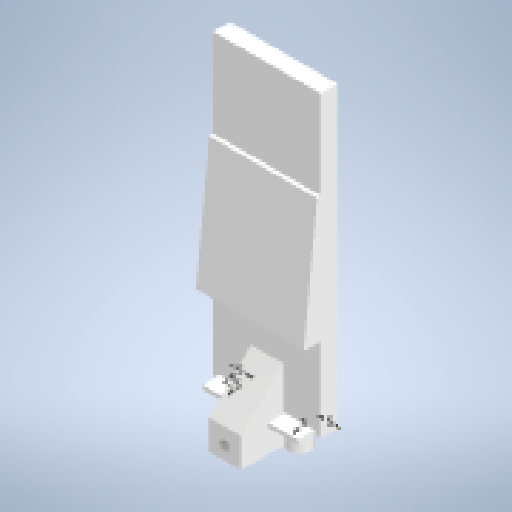
# Autodesk Inventor part: SchubstangeA
Saved by Autodesk Inventor 2025 (Build 290162010, 162A)
## iProperties
Created: 2024-11-26
Part Number: SchubstangeA
Material: PC/ABS-Kunststoff, 3DDruck, PLA
Document SubType Name: Modeling
Designer: Admin
Density: 1.1 g/cm^3
Appearance: Glatt - Weiß(2)
Author: Admin
Autodesk Inventor part; units mm, degrees
ref_plane "YZ Plane" through (0, 0, 0) normal (1, 0, 0) x (0, 1, 0)
ref_plane "XZ Plane" through (0, 0, 0) normal (0, 1, 0) x (-1, 0, 0)
ref_plane "XY Plane" through (0, 0, 0) normal (0, 0, 1) x (1, 0, 0)
sketch "Skizze1" plane through (0, 0, 0) normal (0, 1, 0) x (-1, 0, 0)
  line L0 (16.6592, -105.2226) -> (-8.9408, -105.2226)
  line L1 (-8.9408, -105.2226) -> (-8.9408, -28.2226)
  line L2 (16.6592, -28.2226) -> (16.6592, -105.2226)
  line L3 (3.8592, 157.3916) -> (3.8592, -262.6084)
  line L4 (16.6592, -28.2226) -> (-8.9408, -28.2226)
  line L5 (-8.9408, -105.2226) -> (0.0592, -105.2226)
  line L6 (0.0592, -105.2226) -> (0.0592, -99.2226)
  line L7 (0.0592, -99.2226) -> (-8.9408, -99.2226)
  line L8 (-8.9408, -99.2226) -> (-8.9408, -105.2226)
  line L9 (16.6592, -105.2226) -> (7.6592, -105.2226)
  line L10 (7.6592, -105.2226) -> (7.6592, -99.2226)
  line L11 (7.6592, -99.2226) -> (16.6592, -99.2226)
  line L12 (16.6592, -99.2226) -> (16.6592, -105.2226)
  point P0 (0, 0)
  point P1 (3.8592, -105.2226)
  point P2 (0.0592, -105.2226)
  point P3 (7.6592, -105.2226)
  dimension "d9" = 25.6
  dimension "d48" = 77
  dimension "d49" = 9
  dimension "d50" = 6
  dimension "d51" = 9
  dimension "d52" = 6
  constraints: 26 end point, 5 parallel, 3 horizontal, 3 perpendicular, 1 midpoint, 1 point on line, 1 vertical, 3 other
  measures "d9" distance of L0.start L0.end
  measures "d48" distance between parallel lines of L4 L0
  measures "d49" distance of L7.end L6.end
  measures "d50" distance of L6.end L5.end
  measures "d51" distance of L10.end L11.end
  measures "d52" distance of L9.end L10.end
extrude "Extrusion1" add sketch "Skizze1" along normal blind 4 contours L0 L3 L4 L2 L11 L10 | L0 L6 L7 L1 L4 L3
sketch "Skizze3" plane through (1.1408, 0, -99.2226) normal (0, 0, -1) x (-1, 0, 0)
  line L0 (-2.8, 4) -> (-2.8, 0)
  circle A0 centre (-2.8, 0) radius 2.5
  line L1 (12.8, 4) -> (12.8, 0)
  circle A1 centre (12.8, 0) radius 2.5
  line L2 (8.8, 4) -> (17.8, 4) projected
  line L3 (-7.8, 4) -> (1.2, 4) projected
  line L4 (-2.8, 0) -> (12.8, 0)
  dimension "d29" = 5
  dimension "d54" = 5
  dimension "d66" = 4
  dimension "d69" = 5
  dimension "d70" = 5
  constraints: 8 end point, 2 centre point, 2 point on line, 2 vertical, 1 horizontal
  measures "d29" diameter of A0
  measures "d54" diameter of A1
  measures "d66" distance from line of L1.end L2
  measures "d69" distance from line of L2.end L1
  measures "d70" distance from line of L3.start L0
extrude "Extrusion2" add sketch "Skizze3" along normal blind 4
sketch "Skizze4" plane through (0, 0, 0) normal (0, -1, 0) x (1, 0, 0)
  line L0 (8.9408, -28.2226) -> (8.9408, -99.2226) projected
  line L1 (-16.6592, -89.2226) -> (8.9408, -89.2226)
  line L2 (8.9408, -89.2226) -> (8.9408, -49.2226)
  line L3 (8.9408, -49.2226) -> (-16.6592, -49.2226)
  line L4 (-16.6592, -49.2226) -> (-16.6592, -89.2226)
  line L5 (-16.6592, -99.2226) -> (-16.6592, -28.2226) projected
  line L6 (-0.0592, -105.2226) -> (-7.6592, -105.2226) projected
  point P0 (0, 0)
  point P1 (8.9408, -89.2226)
  dimension "d34" = 40
  dimension "d57" = 16
  constraints: 8 end point, 2 parallel, 1 collinear, 1 horizontal, 1 perpendicular, 1 point on line
  measures "d34" distance of L2.end L1.end
  measures "d57" distance between parallel lines of L6 L1
extrude "Extrusion3" add sketch "Skizze4" along normal blind 5
chamfer "Fasen1" distance 40 distance2 4 1 edges at (-3.8592, -5, -49.2226) measured on face at (-3.8592, -5, -49.7226)
sketch "Skizze5" plane through (8.9408, 0, -89.2226) normal (0, 0, -1) x (-1, 0, 0)
  line L0 (0, 0) -> (25.6, 0) projected
  line L1 (0, 0) -> (0, -5) projected
  line L2 (25.6, -5) -> (0, -5) projected
  line L3 (25.6, 0) -> (25.6, -5) projected
  point P0 (8.9408, 0)
extrude "Extrusion4" cut sketch "Skizze5" against normal blind 10
sketch "Skizze6" plane through (0, 0, 0) normal (0, -1, 0) x (1, 0, 0)
  line L0 (-7.6592, -99.2226) -> (-16.6592, -99.2226) projected
  line L1 (-15.1592, -99.2226) -> (-8.1592, -99.2226)
  line L2 (-8.1592, -99.2226) -> (-8.1592, -98.2226)
  line L3 (-8.1592, -98.2226) -> (-15.1592, -98.2226)
  line L4 (-15.1592, -98.2226) -> (-15.1592, -99.2226)
  line L5 (8.9408, -99.2226) -> (-0.0592, -99.2226) projected
  line L6 (7.4408, -99.2226) -> (0.4408, -99.2226)
  line L7 (0.4408, -99.2226) -> (0.4408, -98.2226)
  line L8 (0.4408, -98.2226) -> (7.4408, -98.2226)
  line L9 (7.4408, -98.2226) -> (7.4408, -99.2226)
  line L10 (1.4408, -99.2226) -> (6.4408, -99.2226) projected
  line L11 (-14.1592, -99.2226) -> (-9.1592, -99.2226) projected
  point P0 (0, 0)
  point P1 (6.4408, -99.2226)
  point P2 (-9.1592, -99.2226)
  point P3 (3.9408, -99.2226)
  point P4 (-11.6592, -99.2226)
  dimension "d60" = 7
  dimension "d61" = 1
  dimension "d62" = 7
  dimension "d63" = 1
  constraints: 16 end point, 4 midpoint, 4 parallel, 2 horizontal, 2 perpendicular, 2 point on line
  measures "d60" distance of L3.end L2.end
  measures "d61" distance of L2.end L1.end
  measures "d62" distance of L7.end L8.end
  measures "d63" distance of L6.end L7.end
extrude "Extrusion5" add sketch "Skizze6" along normal blind 4
sketch "Skizze7" plane through (0, 0, 0) normal (0, -1, 0) x (1, 0, 0)
  line L0 (-0.0592, -99.2226) -> (-0.0592, -105.2226) projected
  line L1 (-0.0592, -105.2226) -> (-7.6592, -105.2226)
  line L2 (-7.6592, -105.2226) -> (-7.6592, -98.2226)
  line L3 (-7.6592, -98.2226) -> (-0.0592, -98.2226)
  line L4 (-0.0592, -98.2226) -> (-0.0592, -105.2226)
  line L5 (-7.6592, -105.2226) -> (-7.6592, -99.2226) projected
  point P0 (0, 0)
  dimension "d71" = 7
  constraints: 8 end point, 2 parallel, 1 collinear, 1 horizontal, 1 perpendicular
  measures "d71" distance of L1.end L2.end
extrude "Extrusion6" add sketch "Skizze7" along normal blind 10
sketch "Skizze2" plane through (0, -10, 0) normal (0, 1, 0) x (1, 0, 0)
  line L0 (8.9408, 28.2226) -> (8.9408, 99.2226) construction
  line L1 (-16.6592, 99.2226) -> (-16.6592, 28.2226) construction
  line L2 (-0.0592, 105.2226) -> (-7.6592, 105.2226) projected
  line L3 (-3.8592, 102.2226) -> (-3.8592, 105.2226)
  point P0 (0, 0)
  point P1 (-16.6592, 28.2226)
  point P2 (8.9408, 106.2444)
  point P3 (-6.8592, 106.2444)
  point P4 (-0.8592, 16.2444)
  point P5 (-6.8592, 16.2444)
  point P6 (-16.6592, 106.2444)
  point P7 (8.9408, 105.2226)
  point P8 (-16.6592, 105.2226)
  point P9 (8.9408, 99.2226)
  point P10 (-3.8592, 103.7226)
  dimension "d53" = 3
  constraints: 2 end point, 2 midpoint, 1 vertical, 2 other
  measures "d53" distance of L3.end L3.start
hole "Bohrung1" at (-3.8592, -10, -102.2226) direction (0, 1, 0) diameter 2.459 end through all thread size "M3x0.5" class "6H" standard "ANSI Metric M Profile"
chamfer "Fasen2" distance 10 angle 45 1 edges at (-3.8592, 0, -98.2226)
